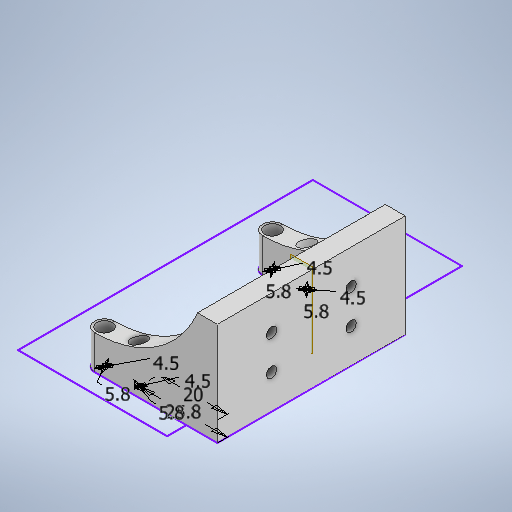
# Autodesk Inventor part: SERVO_TO_TOOLHEAD
Saved by Autodesk Inventor 2025.1 (Build 291241000, 241)
## iProperties
Created: 2024-11-04
Part Number: SERVO_TO_TOOLHEAD
Material: Generic
Document SubType Name: Modeling
Designer: m_kni
Density: 1 g/cm^3
Appearance: Default
Author: m_kni
Autodesk Inventor part; units mm, degrees
ref_plane "YZ Plane" through (0, 0, 0) normal (1, 0, 0) x (0, 1, 0)
ref_plane "XZ Plane" through (0, 0, 0) normal (0, 1, 0) x (-1, 0, 0)
ref_plane "XY Plane" through (0, 0, 0) normal (0, 0, 1) x (1, 0, 0)
sketch "Sketch1" plane through (0, 0, 0) normal (0, 1, 0) x (-1, 0, 0)
  circle A0 centre (-5, -14.4525) radius 2.25
  circle A1 centre (5, -14.4525) radius 2.25
  circle A2 centre (5, 34.5475) radius 2.25
  circle A3 centre (-5, 34.5475) radius 2.25
  line L0 (21.75, 43.0475) -> (-21.75, 43.0475)
  line L1 (21.75, -42.9525) -> (21.75, 43.0475)
  line L2 (-21.75, 43.0475) -> (-21.75, -42.9525)
  line L3 (-21.75, 43.0475) -> (21.75, 43.0475)
  line L4 (21.75, 43.0475) -> (21.75, -42.9525)
  line L5 (21.75, -42.9525) -> (-21.75, -42.9525)
  line L6 (-21.75, -42.9525) -> (-21.75, 43.0475)
  circle A4 centre (-5, 34.5475) radius 2.9
  circle A5 centre (5, 34.5475) radius 2.9
  circle A6 centre (-5, -14.4525) radius 2.9
  circle A7 centre (5, -14.4525) radius 2.9
  line L7 (5, 37.4475) -> (-5, 37.4475)
  line L8 (5, 31.6475) -> (-5, 31.6475)
  line L9 (5, -11.5525) -> (-5, -11.5525)
  line L10 (5, -17.3525) -> (-5, -17.3525)
  line L11 (-5, 37.4475) -> (-30.8, 37.4475)
  line L12 (-5, -17.3525) -> (-30.8, -17.3525)
  line L13 (-30.8, -17.3525) -> (-30.8, 37.4475)
  line L14 (-5, 31.6475) -> (-25, 31.6475)
  line L15 (-25, 31.6475) -> (-25, -11.5525)
  line L16 (-25, -11.5525) -> (-5, -11.5525)
  point P0 (0, 0)
  point P1 (-1.4735, -1.6316)
  dimension "d0" = 5.8
  dimension "d1" = 5.8
  dimension "d2" = 5.8
  dimension "d3" = 5.8
  dimension "d4" = 4.5
  dimension "d5" = 4.5
  dimension "d6" = 4.5
  dimension "d7" = 4.5
  dimension "d8" = 25.8
  dimension "d9" = 20
  constraints: 34 end point, 8 centre point, 8 point on circle, 5 parallel, 5 perpendicular, 4 coincident, 4 horizontal, 2 tangent
  measures "d0" diameter of A4
  measures "d1" diameter of A5
  measures "d2" diameter of A6
  measures "d3" diameter of A7
  measures "d4" diameter of A2
  measures "d5" diameter of A3
  measures "d6" diameter of A0
  measures "d7" diameter of A1
  measures "d8" distance of L7.end L11.end
  measures "d9" distance of L8.end L14.end
extrude "Extrusion1" add sketch "Sketch1" along normal blind 10 contours L11 A4 L14 L2 | L2 L14 L15 L16 L12 L13 L11 | L7 A5 L8 A4 | A4 | L2 L16 A6 L12 | A5 | A6 | A6 L9 A7 L10 | A7
sketch "Sketch2" plane through (25, 0, -11.5525) normal (-1, 0, 0) x (0, 0, 1)
  line L0 (0, 0) -> (0, 10) projected
  line L1 (43.2, 0) -> (43.2, 10) projected
  line L2 (0, 10) -> (43.2, 10)
  line L3 (43.2, 10) -> (43.2, 30)
  line L4 (43.2, 30) -> (0, 30)
  line L5 (0, 30) -> (0, 10)
  point P0 (11.5525, 0)
  dimension "d12" = 20
  constraints: 8 end point, 2 parallel, 1 horizontal, 1 perpendicular
  measures "d12" distance of L3.end L2.end
extrude "Extrusion2" add sketch "Sketch2" against normal up to surface (5.8 mm away)
sketch "Sketch3" plane through (25, 0, -11.5525) normal (-1, 0, 0) x (0, 0, 1)
  line L0 (0, 0) -> (43.2, 0) projected
  line L1 (43.2, 0) -> (43.2, 10) projected
  line L2 (43.2, 10) -> (43.2, 30) projected
  line L3 (43.2, 30) -> (0, 30) projected
  line L4 (0, 30) -> (0, 10) projected
  line L5 (0, 0) -> (0, 10) projected
  circle A0 centre (10, 10) radius 2.75
  line L6 (0, 30) -> (43.2, 30)
  line L7 (43.2, 30) -> (43.2, 0)
  line L8 (43.2, 0) -> (0, 0)
  line L9 (0, 0) -> (0, 30)
  circle A1 centre (10, 20) radius 2.75
  circle A2 centre (33.2, 20) radius 2.75
  circle A3 centre (33.2, 10) radius 2.75
  point P0 (11.5525, 0)
  dimension "d15" = 5.5
  dimension "d16" = 10
  dimension "d17" = 10
  dimension "d18" = 5.5
  dimension "d19" = 5.5
  dimension "d20" = 10
  dimension "d21" = 5.5
  dimension "d22" = 43.2
  dimension "d23" = 30
  constraints: 8 end point, 4 centre point, 2 parallel, 1 horizontal, 1 perpendicular
  measures "d15" diameter of A0
  measures "d16" distance from line of A0.centre L4
  measures "d17" distance from line of A0.centre L0
  measures "d18" diameter of A1
  measures "d19" diameter of A2
  measures "d20" distance from line of L2 A2.centre
  measures "d21" diameter of A3
  measures "d22" distance of L2.end L3.end
  measures "d23" distance of L0.start L3.end
extrude "Extrusion3" cut sketch "Sketch3" against normal blind 3.2 contours A0 | A1 | A2 | A3
sketch "Sketch4" plane through (25, 0, -11.5525) normal (-1, 0, 0) x (0, 0, 1)
  circle A0 centre (10, 10) radius 2.75 projected
  circle A1 centre (10, 10) radius 1.5
  circle A2 centre (10, 20) radius 2.75 projected
  circle A3 centre (10, 20) radius 1.5
  circle A4 centre (33.2, 10) radius 2.75 projected
  circle A5 centre (33.2, 20) radius 2.75 projected
  circle A6 centre (33.2, 10) radius 1.5
  circle A7 centre (33.2, 20) radius 1.5
  point P0 (11.5525, 0)
  dimension "d26" = 3
  dimension "d27" = 3
  dimension "d28" = 3
  dimension "d29" = 3
  constraints: 4 centre point, 4 coincident
  measures "d26" diameter of A1
  measures "d27" diameter of A3
  measures "d28" diameter of A6
  measures "d29" diameter of A7
extrude "Extrusion4" cut sketch "Sketch4" against normal blind 10 contours A1 | A3 | A6 | A7
sketch "Sketch5" plane through (25, 10, 31.6475) normal (0, 0, 1) x (1, 0, 0)
  line L0 (3.2, 7.25) -> (3.2, 12.75) projected
  line L1 (5.8, 0) -> (5.8, 20) projected
  line L2 (0, 20) -> (5.8, 20) projected
  line L3 (0, 0) -> (0, 20) projected
  line L4 (5.8, 0) -> (0, 0) projected
  line L5 (-30, -10) -> (5.8, -10) projected
  line L6 (5.8, -10) -> (5.8, 0) projected
  line L7 (-30, 0) -> (5.8, 0) projected
  line L8 (-30, -10) -> (-30, 0) projected
  line L9 (-30, -10) -> (-30, 0) projected
  arc A0 (-30, 0) -> (0, 20) centre (-30, 32.5) ccw
  line L10 (-30, 0) -> (5.8, 0) projected
  line L11 (-30, 0) -> (0, 0)
  line L12 (-32.9, -10) -> (-32.9, 0) projected
  line L13 (0, 20) -> (0, 0)
  point P0 (-25, -10)
  constraints: 4 end point, 2 point on circle, 2 tangent, 1 centre point, 1 collinear, 1 perpendicular
extrude "Extrusion5" add sketch "Sketch5" along normal up to surface (5.8 mm away) contours L4 L3 L2 L1 | L7 A0 L3
ref_plane "Work Plane1" through (25, 10, 10.0475) normal (0, 0, -1) x (-1, 0, 0)
mirror "Mirror1" about plane through (25, 10, 10.0475) normal (0, 0, -1) of "Extrusion5"
extrude "Extrusion6" cut sketch "Sketch1" along normal blind 33.8125 contours A0 | A1 | A2 | A3
body "Solid1"
